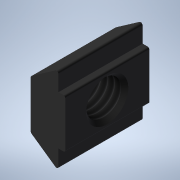
# Autodesk Inventor part: HNTTSS5-5
Saved by Autodesk Inventor 2021 (Build 250183000, 183)
## iProperties
Category: PARTsolutions
Company: MISUMI
Created: 2025-07-19
Part Number: HNTTSS5-5
Material: Generic
Catalog Web Link: www.cadenas.de
Description: HNTT5, HNTTV5, HNTTZ5, HNTTSN5, HNTTSS5-Pre-Assembly Insertion Nuts for Aluminum Extrusions - Standard -For HFS5 Series Aluminum Extrusions 20, 25, 40 Square-
Vendor: MISUMI
Document SubType Name: Modeling
Designer: psAdmin
Manufacturer: MISUMI
Mass: 0.255285 g
Surface Area: 3.31874 cm^2
Volume: 0.255285 cm^3
Density: 1 g/cm^3
Appearance: PSOLRGB-175-175-175
PSOL_IDENT_0: {$CADENAS_DATA/23d-libs/misumi/metric/38_al_extrusions_blackets/nuts/hntt5.prj},193 {VTYP=3D},{NB=HN
PSOL_IDENT_1: TTSS5-5},{LINA=HNTTSS5-5},{NN=HNTT5, HNTTV5, HNTTZ5, HNTTSN5, HNTTSS5},{DATE=16.05.2023 02:29:53},{G
PSOL_IDENT_2: EOMDATE=26.07.2016 05:42:00},{VERSION=},{LINEID=110},{WBVAR=M},{WBNUMERIC=}  {NB=HNTTSS5-5},{LINA=HN
PSOL_IDENT_3: TTSS5-5},{KT=DUMMY},{PN=HNTTSS5-5},{TYPE=HNTTSS5},{MAT=303 Stainless Steel},{M=5},{MALG= '5' },{M3D=
PSOL_IDENT_4: 5},{A=5.8},{B=10.0},{E=3.3},{T=4.1},{L=10},{TT=5.8},{TAPER=3.000}
NB: HNTTSS5-5
NN: HNTT5, HNTTV5, HNTTZ5, HNTTSN5, HNTTSS5
NT: Pre-Assembly Insertion Nuts for Aluminum Extrusions - Standard -For HFS5 Series Aluminum Extrusions 20, 25, 40 Square-
NBSYN: $PN.
LINA: HNTTSS5-5
CATALOG: Misumi
PN: HNTTSS5-5
MAT: 303 Stainless Steel
M: 5
E: 3.3
T: 4.1
SUPPLIER: MISUMI
ARTICLENO: HNTTSS5-5
BOMINFO: HNTTSS5-5
CREATOR: CADENAS GmbH
Title: HNTTSS5-5
Author: Cadenas PARTsolutions
Comments: Pre-Assembly Insertion Nuts for Aluminum Extrusions - Standard -For HFS5 Series Aluminum Extrusions 20, 25, 40 Square-
Autodesk Inventor part; units mm, degrees
sketch "Sketch_2" plane through (0, 0, 0) normal (0, 0, 1) x (1, 0, 0)
  arc A0 (-4.1, -2.7438) -> (-3.972, -2.9896) centre (-3.8, -2.7438) ccw
  line L0 (-3.972, -2.9896) -> (-1.1589, -4.9588)
  arc A1 (-1.1589, -4.9588) -> (-0.8, -4.7719) centre (-1.0281, -4.7719) ccw
  line L1 (-0.8, -4.7719) -> (-0.8, -2.9)
  line L2 (-0.8, -2.9) -> (-0.2, -2.9)
  arc A2 (-0.2, -2.9) -> (0, -2.7) centre (-0.2, -2.7) ccw
  line L3 (0, -2.7) -> (0, 2.7)
  arc A3 (0, 2.7) -> (-0.2, 2.9) centre (-0.2, 2.7) ccw
  line L4 (-0.2, 2.9) -> (-0.8, 2.9)
  line L5 (-0.8, 2.9) -> (-0.8, 4.7719)
  arc A4 (-0.8, 4.7719) -> (-1.1589, 4.9588) centre (-1.0281, 4.7719) ccw
  line L6 (-1.1589, 4.9588) -> (-3.972, 2.9896)
  arc A5 (-3.972, 2.9896) -> (-4.1, 2.7438) centre (-3.8, 2.7438) ccw
  line L7 (-4.1, 2.7438) -> (-4.1, -2.7438)
  constraints: 16 end point, 12 point on circle, 6 centre point
extrude "Extrusion1" add sketch "Sketch_2" along normal mid plane 10
sketch "Sketch_5" plane through (0, 0, 0) normal (0, 0, 1) x (1, 0, 0)
  line L0 (0, 0) -> (-4.1, 0)
  line L1 (-4.1, 0) -> (-4.1, 2.5)
  line L2 (-4.1, 2.5) -> (-3.667, 2.067)
  line L3 (-3.667, 2.067) -> (-0.433, 2.067)
  line L4 (-0.433, 2.067) -> (0, 2.5)
  line L5 (0, 2.5) -> (0, 0)
  line L6 (0, 0) -> (-4.1, 0)
  constraints: 14 end point
revolve "Revolution1" cut sketch "Sketch_5" angle 360 about axis through (0, 0, 0) along (1, 0, 0)
thread "Thread1" size "M5x0.8" class "6H" standard "ISO Metric profile" full length
ref_plane "nut_XY" through (0, 0, 0) normal (1, 0, 0) x (0, 0, -1)
ref_plane "nut_YZ" through (0, 0, 0) normal (0, 0, -1) x (0, 1, 0)
ref_plane "nut_ZX" through (0, 0, 0) normal (0, 1, 0) x (1, 0, 0)
ref_plane "to_bolt_XY" through (-4.1, 0, 0) normal (1, 0, 0) x (0, 0, -1)
ref_plane "to_bolt_YZ" through (-4.1, 0, 0) normal (0, 0, -1) x (0, 1, 0)
ref_plane "to_bolt_ZX" through (-4.1, 0, 0) normal (0, 1, 0) x (1, 0, 0)
ref_plane "to_frames_XY" through (-0.8, 0, 0) normal (1, 0, 0) x (0, 0, -1)
ref_plane "to_frames_YZ" through (-0.8, 0, 0) normal (0, 0, -1) x (0, 1, 0)
ref_plane "to_frames_ZX" through (-0.8, 0, 0) normal (0, 1, 0) x (1, 0, 0)
ref_plane "to_lane_XY" through (0, 0, 0) normal (0, 0, 1) x (1, 0, 0)
ref_plane "to_lane_YZ" through (0, 0, 0) normal (1, 0, 0) x (0, 1, 0)
ref_plane "to_lane_ZX" through (0, 0, 0) normal (0, 1, 0) x (0, 0, 1)
body "Solid1"
